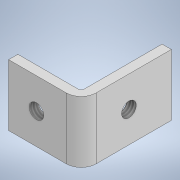
# Autodesk Inventor part: Threaded Right Support Farnell1466885
Saved by Autodesk Inventor 2021 (Build 250183000, 183)
## iProperties
Created: 2020-08-04
Part Number: Threaded Right Support Farnell1466885
Material: Generic
Document SubType Name: Modeling
Designer: jgray
Density: 1 g/cm^3
Appearance: Default
Author: jgray
Autodesk Inventor part; units mm, degrees
ref_plane "YZ Plane" through (0, 0, 0) normal (1, 0, 0) x (0, 1, 0)
ref_plane "XZ Plane" through (0, 0, 0) normal (0, 1, 0) x (-1, 0, 0)
ref_plane "XY Plane" through (0, 0, 0) normal (0, 0, 1) x (1, 0, 0)
sketch "Sketch1" plane through (0, 0, 0) normal (0, 1, 0) x (-1, 0, 0)
  line L0 (0, 0) -> (12.16, 0)
  line L1 (12.16, 0) -> (12.16, -1.55)
  line L2 (1.55, -15.12) -> (0, -15.12)
  line L3 (0, -15.12) -> (0, 0)
  line L4 (10.61, -1.55) -> (1.55, -1.55)
  line L5 (1.55, -1.55) -> (1.55, -13.57)
  line L6 (10.61, -1.55) -> (12.16, -1.55)
  line L7 (1.55, -13.57) -> (1.55, -15.12)
  dimension "d2" = 1.55
  dimension "d3" = 12.16
  dimension "d4" = 15.12
  constraints: 16 end point, 2 horizontal, 2 parallel, 2 perpendicular, 1 other
  measures "d2" distance between parallel lines of L0 L4
  measures "d3" distance between parallel lines of L3 L1
  measures "d4" distance of L2.end L0.start
extrude "Extrusion1" add sketch "Sketch1" along normal blind 10.3
sketch "Sketch2" plane through (-12.16, 0, 0) normal (0, 0, 1) x (1, 0, 0)
  line L0 (4.66, 14.5613) -> (4.66, -2.7265)
  line L1 (12.16, 0) -> (12.16, 10.3) projected
  line L2 (-7.6119, 5.15) -> (15.8963, 5.15)
  point P0 (12.16, 5.15)
  point P1 (4.66, 5.15)
  dimension "d7" = 7.5
  constraints: 4 end point, 3 point on line, 1 horizontal, 1 midpoint, 1 vertical
  measures "d7" distance between parallel lines of L0 L1
hole "Hole1" at (-7.5, 5.15, 0) direction (0, 0, -1) diameter 2.459 end through all thread size "M3x0.5" class "6H" standard "ANSI Metric M Profile"
sketch "Sketch3" plane through (0, 0, 0) normal (1, 0, 0) x (0, 0, -1)
  line L0 (-10.3606, 5.15) -> (23.1245, 5.15)
  line L1 (8, 14.2786) -> (8, -6.8061)
  line L2 (0, 0) -> (0, 10.3) projected
  point P0 (0, 5.15)
  point P1 (8, 5.15)
  dimension "d15" = 8
  constraints: 4 end point, 3 point on line, 1 horizontal, 1 midpoint, 1 vertical
  measures "d15" distance between parallel lines of L1 L2
hole "Hole2" at (0, 5.15, -8) direction (-1, 0, 0) diameter 2.459 end through all thread size "M3x0.5" class "6H" standard "ANSI Metric M Profile"
fillet "Fillet1" radius 2.5 1 edges at (0, 5.15, 0)
fillet "Fillet2" radius 0.5 1 edges at (-1.55, 5.15, -1.55)
body "Solid1"
